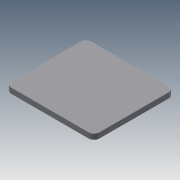
# Autodesk Inventor part: HbSensorCover01
Saved by Autodesk Inventor 2015 SP1 (Build 190203100, 203)
## iProperties
Created: 2015-11-01
Part Number: HbSensorCover01
Material: Generic
Document SubType Name: Modeling
Designer: Yamaura
Density: 1 g/cm^3
Appearance: Default
Author: Yamaura
Autodesk Inventor part; units mm, degrees
ref_plane "YZ Plane" through (0, 0, 0) normal (1, 0, 0) x (0, 1, 0)
ref_plane "XZ Plane" through (0, 0, 0) normal (0, 1, 0) x (-1, 0, 0)
ref_plane "XY Plane" through (0, 0, 0) normal (0, 0, 1) x (1, 0, 0)
sketch "スケッチ1" plane through (0, 0, 0) normal (0, 1, 0) x (-1, 0, 0)
  line L0 (-16.5, 15) -> (16.5, 15)
  line L1 (16.5, 15) -> (16.5, -15)
  line L2 (16.5, -15) -> (-16.5, -15)
  line L3 (-16.5, -15) -> (-16.5, 15)
  line L4 (-16.5, 15) -> (16.5, -15) construction
  line L5 (16.5, 15) -> (-16.5, -15) construction
  point P0 (0, 0)
  dimension "d0" = 33
  dimension "d1" = 30
  constraints: 12 end point, 2 midpoint, 2 parallel, 1 horizontal, 1 perpendicular
  measures "d0" distance of L1.end L2.end
  measures "d1" distance of L0.end L1.end
extrude "押し出し1" add sketch "スケッチ1" along normal blind 2
fillet "フィレット1" radius 2 4 edges at (16.5, 1, 15) (16.5, 1, -15) (-16.5, 1, 15) (-16.5, 1, -15)
